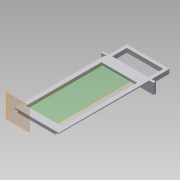
# Autodesk Inventor part: 41_Objektträger_Tray
Saved by Autodesk Inventor 2015 (Build 190159000, 159)
## iProperties
Created: 2015-04-03
Part Number: 41_Objektträger_Tray
Material: Generisch
Document SubType Name: Modeling
Designer: Bene
Density: 1 g/cm^3
Appearance: Weiß
Author: Bene
Autodesk Inventor part; units mm, degrees
ref_plane "YZ Plane" through (0, 0, 0) normal (1, 0, 0) x (0, 1, 0)
ref_plane "XZ Plane" through (0, 0, 0) normal (0, 1, 0) x (-1, 0, 0)
ref_plane "XY Plane" through (0, 0, 0) normal (0, 0, 1) x (1, 0, 0)
ref_plane "Arbeitsebene1" through (-10.2983, 3.243, -1) normal (0, 0, -1) x (-1, 0, 0)
sketch "Skizze1" plane through (-10.2983, 3.243, -1) normal (0, 0, -1) x (-1, 0, 0)
  line L0 (2.7017, 34.757) -> (-23.2983, 34.757) projected
  line L1 (-23.2983, 34.757) -> (-23.2983, -41.243) projected
  line L2 (-23.2983, -41.243) -> (2.7017, -41.243) projected
  line L3 (2.7017, -41.243) -> (2.7017, 34.757) projected
  line L4 (3.7017, -42.243) -> (-24.2983, -42.243)
  line L5 (-24.2983, -42.243) -> (-24.2983, 35.757)
  line L6 (-24.2983, 35.757) -> (3.7017, 35.757)
  line L7 (3.7017, 35.757) -> (3.7017, -42.243)
  line L8 (7.7017, -46.243) -> (-28.2983, -46.243)
  line L9 (-28.2983, -46.243) -> (-28.2983, 39.757)
  line L10 (-28.2983, 39.757) -> (7.7017, 39.757)
  line L11 (7.7017, 39.757) -> (7.7017, -46.243)
  point P0 (-10.2983, -3.243)
  dimension "d1" = 4
  dimension "d39" = 36
  constraints: 16 end point, 6 other
  measures "d1" distance between parallel lines of L7 L11
  measures "d39" distance between parallel lines of L11 L9
extrude "Extrusion1" add sketch "Skizze1" along normal blind 3 contours L8 L9 L10 L11
sketch "Skizze2" plane through (-10.2983, 3.243, -1) normal (0, 0, 1) x (1, 0, 0)
  line L0 (24.2983, 35.757) -> (24.2983, -42.243) projected
  line L1 (24.2983, -42.243) -> (-3.7017, -42.243) projected
  line L2 (-3.7017, -42.243) -> (-3.7017, 35.757) projected
  line L3 (-3.7017, 35.757) -> (24.2983, 35.757) projected
  line L4 (-7.7017, -46.243) -> (28.2983, -46.243) projected
  line L5 (28.2983, -46.243) -> (28.2983, 39.757) projected
  line L6 (28.2983, 39.757) -> (-7.7017, 39.757) projected
  line L7 (-7.7017, 39.757) -> (-7.7017, -46.243) projected
  line L8 (22.2983, 33.757) -> (22.2983, -40.243)
  line L9 (22.2983, -40.243) -> (-1.7017, -40.243)
  line L10 (-1.7017, -40.243) -> (-1.7017, 33.757)
  line L11 (-1.7017, 33.757) -> (22.2983, 33.757)
  line L12 (21.2983, -39.243) -> (21.2983, 32.757)
  line L13 (21.2983, 32.757) -> (-0.7017, 32.757)
  line L14 (-0.7017, 32.757) -> (-0.7017, -39.243)
  line L15 (-0.7017, -39.243) -> (21.2983, -39.243)
  point P0 (10.2983, -3.243)
  dimension "d4" = 2
  dimension "d45" = 1
  constraints: 16 end point, 6 other
  measures "d4" distance between parallel lines of L3 L11
  measures "d45" distance between parallel lines of L8 L12
extrude "Extrusion2" add sketch "Skizze2" along normal blind 1 contours L0 L1 L2 L3 | L7 L6 L5 L4 | L8 L9 L10 L11
ref_plane "Arbeitsebene2" through (-18, -43, -2.5) normal (0, -1, 0) x (1, 0, 0)
sketch "Skizze9" plane through (-18, -43, -4) normal (-1, 0, 0) x (0, 0, 1)
  line L0 (0, 86) -> (4, 86) projected
  line L1 (0, 0) -> (0, 86) projected
  line L2 (4, 0) -> (0, 0) projected
  line L3 (4, 86) -> (4, 0) projected
  line L4 (4, 0) -> (3, 0)
  line L5 (3, 0) -> (3, 86)
  line L6 (3, 86) -> (4, 86)
  line L7 (4, 86) -> (4, 0)
  line L8 (4, 0) -> (3, 86) construction
  line L9 (3, 0) -> (4, 86) construction
  dimension "d27" = 1
  constraints: 12 end point, 2 parallel, 1 horizontal, 1 perpendicular, 1 point on line
  measures "d27" distance of L0.end L5.end
extrude "Extrusion9" add sketch "Skizze9" along normal blind 3 contours L0 L3 L2 L5
sketch "Skizze10" plane through (18, -43, -4) normal (1, 0, 0) x (0, 0, -1)
  line L0 (-3, 86) -> (-3, 0) projected
  line L1 (-3, 0) -> (-4, 0) projected
  line L2 (-4, 0) -> (-4, 86) projected
  line L3 (-4, 86) -> (-3, 86) projected
  point P0 (-4, 43)
extrude "Extrusion10" add sketch "Skizze10" along normal blind 3
sketch "Skizze11" plane through (-10.2983, 3.243, 0) normal (0, 0, 1) x (1, 0, 0)
  line L0 (22.2983, -40.243) -> (-1.7017, -40.243) projected
  line L1 (-1.7017, -40.243) -> (-1.7017, 33.757) projected
  line L2 (-1.7017, 33.757) -> (22.2983, 33.757) projected
  line L3 (22.2983, 33.757) -> (22.2983, -40.243) projected
  line L4 (31.2983, 39.757) -> (-9.4351, 39.757)
  line L5 (-9.4351, 39.757) -> (-9.4351, 59.757)
  line L6 (-9.4351, 59.757) -> (31.2983, 59.757)
  line L7 (31.2983, 59.757) -> (31.2983, 39.757)
  line L8 (28.2983, 42.757) -> (-6.4351, 42.757)
  line L9 (-6.4351, 42.757) -> (-6.4351, 56.757)
  line L10 (-6.4351, 56.757) -> (28.2983, 56.757)
  line L11 (28.2983, 56.757) -> (28.2983, 42.757)
  point P0 (10.2983, -3.243)
  dimension "d32" = 20
  dimension "d33" = 3
  constraints: 16 end point, 4 parallel, 2 perpendicular, 1 horizontal, 3 other
  measures "d32" distance of L4.end L5.end
  measures "d33" distance between parallel lines of L7 L11
extrude "Extrusion11" add sketch "Skizze11" against normal up to surface (4 mm away) contours L4 L5 L6 L7
sketch "Skizze12" plane through (-10.2983, 3.243, 0) normal (0, 0, 1) x (1, 0, 0)
  line L0 (28.2983, 56.757) -> (28.2983, 42.757) projected
  line L1 (28.2983, 42.757) -> (-6.4351, 42.757) projected
  line L2 (-6.4351, 42.757) -> (-6.4351, 56.757) projected
  line L3 (-6.4351, 56.757) -> (28.2983, 56.757) projected
  line L4 (31.2983, -46.243) -> (31.2983, 59.757) projected
  line L5 (31.2983, 59.757) -> (-9.4351, 59.757) projected
  line L6 (-9.4351, 59.757) -> (-9.4351, 39.757) projected
  line L7 (35.2983, 40.5388) -> (-14.7017, 40.5388)
  line L8 (-14.7017, 40.5388) -> (-14.7017, 42.757)
  line L9 (-14.7017, 42.757) -> (35.2983, 42.757)
  line L10 (35.2983, 42.757) -> (35.2983, 40.5388)
  line L11 (35.2983, 40.5388) -> (-14.7017, 42.757) construction
  line L12 (-14.7017, 40.5388) -> (35.2983, 42.757) construction
  line L13 (31.2983, -46.243) -> (-10.7017, -46.243) projected
  line L14 (-10.7017, 39.757) -> (-9.4351, 39.757) projected
  line L15 (-10.7017, -46.243) -> (-10.7017, 39.757) projected
  point P0 (10.2983, -3.243)
  point P1 (10.2983, 41.6479)
  dimension "d36" = 50
  constraints: 12 end point, 2 midpoint, 2 parallel, 1 horizontal, 1 perpendicular, 1 point on line
  measures "d36" distance of L8.end L9.end
extrude "Extrusion12" add sketch "Skizze12" against normal blind 10 contours L9 L4 L7 L6 L1 | L9 L10 L7 L4 | L6 L7 L8 L9
sketch "Skizze13" plane through (-10.2983, 3.243, -4) normal (0, 0, -1) x (-1, 0, 0)
  line L0 (-24.2983, -42.243) -> (-24.2983, 35.757) projected
  line L1 (-24.2983, 35.757) -> (3.7017, 35.757) projected
  line L2 (3.7017, 35.757) -> (3.7017, -42.243) projected
  line L3 (3.7017, -42.243) -> (-24.2983, -42.243) projected
  line L4 (9.4351, 40.5388) -> (-31.2983, 40.5388) projected
  line L5 (-31.2983, 39.757) -> (-31.2983, 40.5388) projected
  line L6 (-28.2983, 39.757) -> (-31.2983, 39.757) projected
  line L7 (-28.2983, 39.757) -> (-28.2983, -46.243) projected
  line L8 (-28.2983, -46.243) -> (7.7017, -46.243) projected
  line L9 (7.7017, -46.243) -> (7.7017, 39.757) projected
  line L10 (9.4351, 39.757) -> (7.7017, 39.757) projected
  line L11 (9.4351, 40.5388) -> (9.4351, 39.757) projected
  line L12 (-27.2983, -42.243) -> (6.7017, -42.243)
  line L13 (6.7017, -42.243) -> (6.7017, 35.757)
  line L14 (6.7017, 35.757) -> (-27.2983, 35.757)
  line L15 (-27.2983, 35.757) -> (-27.2983, -42.243)
  line L16 (-27.2983, -42.243) -> (6.7017, 35.757) construction
  line L17 (6.7017, -42.243) -> (-27.2983, 35.757) construction
  point P0 (-10.2983, -3.243)
  dimension "d40" = 34
  constraints: 12 end point, 2 midpoint, 2 parallel, 1 horizontal, 1 perpendicular
  measures "d40" distance of L14.end L13.end
extrude "Extrusion13" cut sketch "Skizze13" against normal up to surface (3 mm away) contours L12 L15 L14 L0 | L2 L14 L13 L12
sketch "Skizze14" plane through (-10.2983, 3.243, -4) normal (0, 0, -1) x (-1, 0, 0)
  line L0 (6.7017, -42.243) -> (-27.2983, -42.243) projected
  line L1 (-27.2983, -42.243) -> (-27.2983, 35.757) projected
  line L2 (-27.2983, 35.757) -> (6.7017, 35.757) projected
  line L3 (6.7017, 35.757) -> (6.7017, -42.243) projected
  line L4 (9.4351, 40.5388) -> (-31.2983, 40.5388) projected
  line L5 (-31.2983, 39.757) -> (-31.2983, 40.5388) projected
  line L6 (-28.2983, 39.757) -> (-31.2983, 39.757) projected
  line L7 (-28.2983, 39.757) -> (-28.2983, -46.243) projected
  line L8 (-28.2983, -46.243) -> (7.7017, -46.243) projected
  line L9 (7.7017, -46.243) -> (7.7017, 39.757) projected
  line L10 (9.4351, 39.757) -> (7.7017, 39.757) projected
  line L11 (9.4351, 40.5388) -> (9.4351, 39.757) projected
  point P0 (-10.2983, -3.243)
extrude "Extrusion14" cut sketch "Skizze14" against normal blind 1
sketch "Skizze15" plane through (-10.2983, 3.243, -1) normal (0, 0, -1) x (-1, 0, 0)
  line L0 (0.7017, -39.243) -> (-21.2983, -39.243) projected
  line L1 (-21.2983, -39.243) -> (-21.2983, 32.757) projected
  line L2 (-21.2983, 32.757) -> (0.7017, 32.757) projected
  line L3 (0.7017, 32.757) -> (0.7017, -39.243) projected
  line L4 (-27.2983, -42.243) -> (6.7017, -42.243) projected
  line L5 (6.7017, -42.243) -> (6.7017, 35.757) projected
  line L6 (6.7017, 35.757) -> (-27.2983, 35.757) projected
  line L7 (-27.2983, 35.757) -> (-27.2983, -42.243) projected
  line L8 (6.7017, -39.243) -> (-27.2983, -39.243)
  line L9 (-27.2983, -39.243) -> (-27.2983, 32.757)
  line L10 (-27.2983, 32.757) -> (6.7017, 32.757)
  line L11 (6.7017, 32.757) -> (6.7017, -39.243)
  line L12 (6.7017, -39.243) -> (-27.2983, 32.757) construction
  line L13 (-27.2983, -39.243) -> (6.7017, 32.757) construction
  point P0 (-10.2983, -3.243)
  constraints: 12 end point, 2 midpoint, 2 parallel, 1 horizontal, 1 perpendicular, 1 point on line
extrude "Extrusion15" cut sketch "Skizze15" against normal through all contours L3 L10 L5 L8 | L8 L7 L10 L1
